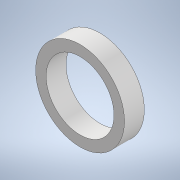
# Autodesk Inventor part: kokool
Saved by Autodesk Inventor 2022.3 (Build 263350000, 350)
## iProperties
Created: 2023-01-15
Part Number: kokool
Material: Generic
Document SubType Name: Modeling
Designer: komputer
Density: 1 g/cm^3
Appearance: Default
Author: komputer
Autodesk Inventor part; units mm, degrees
ref_plane "YZ Plane" through (0, 0, 0) normal (1, 0, 0) x (0, 1, 0)
ref_plane "XZ Plane" through (0, 0, 0) normal (0, 1, 0) x (-1, 0, 0)
ref_plane "XY Plane" through (0, 0, 0) normal (0, 0, 1) x (1, 0, 0)
sketch "Sketch1" plane through (0, 0, 0) normal (0, 0, 1) x (1, 0, 0)
  circle A0 centre (1.5, 0) radius 7 projected
  circle A1 centre (1.5, 0) radius 7 projected
  circle A2 centre (1.5, 0) radius 1.5 projected
  circle A3 centre (1.5, 0) radius 1 projected
  line L0 (16.2929, 8.3594) -> (-3.7046, 8.2678)
  line L1 (1.5, 0) -> (1.462, 8.2914)
  line L2 (1.462, 8.2914) -> (1.4574, 9.2914)
  line L3 (-7.6528, 0.7576) -> (-7.6612, 1.3735) projected
  ellipse E0 centre (-7.4913, -0.0469) end of major axis (-7.487, -1.0469) minor radius 0.015 projected
  ellipse E1 centre (-7.4913, -0.0469) end of major axis (-7.487, -1.0469) minor radius 0.015 projected
  ellipse E2 centre (-7.5641, 0.5606) end of major axis (-7.5648, 0.7606) minor radius 0.0029 (-7.5669, 0.6786) -> (-7.5649, 0.3868) ccw projected
  ellipse E3 centre (-7.607, -0.1095) end of major axis (-7.6033, -1.1095) minor radius 0.0145 projected
  ellipse E4 centre (-7.607, -0.1095) end of major axis (-7.6033, -1.1095) minor radius 0.0145 projected
  ellipse E5 centre (-7.4913, -0.0469) end of major axis (-7.487, -1.0469) minor radius 0.015 projected
  ellipse E6 centre (-7.4369, -0.2282) end of major axis (-7.4378, -0.0282) minor radius 0.003 (-7.4348, -0.4079) -> (-7.4361, -0.0582) ccw projected
  ellipse E7 centre (-7.4913, -0.0469) end of major axis (-7.487, -1.0469) minor radius 0.015 projected
  ellipse E8 centre (-7.4913, -0.0469) end of major axis (-7.487, -1.0469) minor radius 0.015 projected
  ellipse E9 centre (-7.5547, -1.7062) end of major axis (-7.5554, -1.5062) minor radius 0.0029 (-7.5538, -1.906) -> (-7.5527, -1.5926) ccw projected
  ellipse E10 centre (-7.6485, -1.6199) end of major axis (-7.6492, -1.4199) minor radius 0.0029 (-7.6512, -1.502) -> (-7.6479, -1.8195) ccw projected
  line L4 (-7.6369, -1.8711) -> (-7.6479, -1.8195) projected
  ellipse E11 centre (-7.6364, -2.0707) end of major axis (-7.6371, -1.8707) minor radius 0.0029 (-7.6334, -2.1069) -> (-7.6369, -1.8711) ccw projected
  line L5 (-7.6327, -2.8428) -> (-7.6334, -2.1069) projected
  ellipse E12 centre (-7.6297, -2.879) end of major axis (-7.6304, -2.679) minor radius 0.0029 (-7.6327, -2.8428) -> (-7.6279, -3.0648) ccw projected
  line L6 (-7.6189, -2.7874) -> (-7.6279, -3.0648) projected
  ellipse E13 centre (-7.6171, -2.9732) end of major axis (-7.6179, -2.7732) minor radius 0.0029 (-7.6145, -2.9205) -> (-7.6189, -2.7874) ccw projected
  line L7 (-7.609, -3.6423) -> (-7.6145, -2.9205) projected
  ellipse E14 centre (-7.6064, -3.5896) end of major axis (-7.6072, -3.3896) minor radius 0.0029 (-7.609, -3.6423) -> (-7.6038, -3.7248) ccw projected
  line L8 (-7.5985, -3.1734) -> (-7.6038, -3.7248) projected
  ellipse E15 centre (-7.5958, -3.3085) end of major axis (-7.5966, -3.1086) minor radius 0.0029 (-7.5941, -3.1773) -> (-7.5985, -3.1734) ccw projected
  line L9 (-7.585, -3.7421) -> (-7.5941, -3.1773) projected
  ellipse E16 centre (-7.5833, -3.6109) end of major axis (-7.584, -3.4109) minor radius 0.0029 (-7.585, -3.7421) -> (-7.5803, -3.6688) ccw projected
  line L10 (-7.5798, -2.9524) -> (-7.5803, -3.6688) projected
  ellipse E17 centre (-7.5768, -3.0103) end of major axis (-7.5775, -2.8103) minor radius 0.0029 (-7.5763, -2.8266) -> (-7.5798, -2.9524) ccw projected
  line L11 (-7.5652, -3.1224) -> (-7.5763, -2.8266) projected
  ellipse E18 centre (-7.5648, -2.9387) end of major axis (-7.5655, -2.7387) minor radius 0.0029 (-7.5652, -3.1224) -> (-7.562, -2.9078) ccw projected
  line L12 (-7.5664, -2.1685) -> (-7.562, -2.9078) projected
  ellipse E19 centre (-7.5637, -2.1375) end of major axis (-7.5644, -1.9375) minor radius 0.0029 (-7.5645, -1.9377) -> (-7.5664, -2.1685) ccw projected
  line L13 (-7.5538, -1.906) -> (-7.5645, -1.9377) projected
  ellipse E20 centre (-7.5547, -1.7062) end of major axis (-7.5554, -1.5062) minor radius 0.0029 (-7.5538, -1.906) -> (-7.5527, -1.5926) ccw projected
  line L14 (-7.5611, -0.9767) -> (-7.5527, -1.5926) projected
  ellipse E21 centre (-7.5591, -0.8631) end of major axis (-7.5599, -0.6631) minor radius 0.0029 (-7.5612, -0.6867) -> (-7.5611, -0.9767) ccw projected
  line L15 (-7.5529, -0.3338) -> (-7.5612, -0.6867) projected
  ellipse E22 centre (-7.5549, -0.1574) end of major axis (-7.5556, 0.0426) minor radius 0.0029 (-7.5529, -0.3338) -> (-7.5541, 0.0164) ccw projected
  line L16 (-7.5649, 0.3868) -> (-7.5541, 0.0164) projected
  ellipse E23 centre (-7.5641, 0.5606) end of major axis (-7.5648, 0.7606) minor radius 0.0029 (-7.5669, 0.6786) -> (-7.5649, 0.3868) ccw projected
  line L17 (-7.5627, 1.2829) -> (-7.5669, 0.6786) projected
  ellipse E24 centre (-7.5655, 1.4008) end of major axis (-7.5662, 1.6008) minor radius 0.0029 (-7.5627, 1.2829) -> (-7.566, 1.6004) ccw projected
  line L18 (-7.577, 1.652) -> (-7.566, 1.6004) projected
  ellipse E25 centre (-7.5775, 1.8516) end of major axis (-7.5783, 2.0516) minor radius 0.0029 (-7.5805, 1.8878) -> (-7.577, 1.652) ccw projected
  line L19 (-7.5812, 2.6237) -> (-7.5805, 1.8878) projected
  ellipse E26 centre (-7.5842, 2.66) end of major axis (-7.585, 2.86) minor radius 0.0029 (-7.5812, 2.6237) -> (-7.586, 2.8457) ccw projected
  line L20 (-7.595, 2.5683) -> (-7.586, 2.8457) projected
  ellipse E27 centre (-7.5968, 2.7541) end of major axis (-7.5975, 2.9541) minor radius 0.0029 (-7.5994, 2.7014) -> (-7.595, 2.5683) ccw projected
  line L21 (-7.6049, 3.4233) -> (-7.5994, 2.7014) projected
  ellipse E28 centre (-7.6075, 3.3705) end of major axis (-7.6082, 3.5705) minor radius 0.0029 (-7.6049, 3.4233) -> (-7.6101, 3.5057) ccw projected
  line L22 (-7.6154, 2.9543) -> (-7.6101, 3.5057) projected
  ellipse E29 centre (-7.6181, 3.0895) end of major axis (-7.6188, 3.2895) minor radius 0.0029 (-7.6198, 2.9582) -> (-7.6154, 2.9543) ccw projected
  line L23 (-7.629, 3.523) -> (-7.6198, 2.9582) projected
  ellipse E30 centre (-7.6307, 3.3918) end of major axis (-7.6314, 3.5918) minor radius 0.0029 (-7.629, 3.523) -> (-7.6337, 3.4497) ccw projected
  line L24 (-7.6342, 2.7334) -> (-7.6337, 3.4497) projected
  ellipse E31 centre (-7.6372, 2.7912) end of major axis (-7.6379, 2.9912) minor radius 0.0029 (-7.6376, 2.6075) -> (-7.6342, 2.7334) ccw projected
  line L25 (-7.6487, 2.9034) -> (-7.6376, 2.6075) projected
  ellipse E32 centre (-7.6492, 2.7196) end of major axis (-7.6499, 2.9196) minor radius 0.0029 (-7.6487, 2.9034) -> (-7.6519, 2.6887) ccw projected
  line L26 (-7.6475, 1.9494) -> (-7.6519, 2.6887) projected
  ellipse E33 centre (-7.6503, 1.9184) end of major axis (-7.651, 2.1184) minor radius 0.0029 (-7.6494, 1.7186) -> (-7.6475, 1.9494) ccw projected
  line L27 (-7.6601, 1.6869) -> (-7.6494, 1.7186) projected
  ellipse E34 centre (-7.6593, 1.4871) end of major axis (-7.66, 1.6871) minor radius 0.0029 (-7.6601, 1.6869) -> (-7.6612, 1.3735) ccw projected
  line L28 (-7.6528, 0.7576) -> (-7.6612, 1.3735) projected
  ellipse E35 centre (-7.6548, 0.644) end of major axis (-7.6555, 0.844) minor radius 0.0029 (-7.6528, 0.4676) -> (-7.6528, 0.7576) ccw projected
  line L29 (-7.661, 0.1147) -> (-7.6528, 0.4676) projected
  ellipse E36 centre (-7.659, -0.0617) end of major axis (-7.6598, 0.1383) minor radius 0.0029 (-7.661, 0.1147) -> (-7.6598, -0.2354) ccw projected
  line L30 (-7.649, -0.6059) -> (-7.6598, -0.2354) projected
  ellipse E37 centre (-7.6498, -0.7797) end of major axis (-7.6506, -0.5797) minor radius 0.0029 (-7.6471, -0.8977) -> (-7.649, -0.6059) ccw projected
  line L31 (-7.6512, -1.502) -> (-7.6471, -0.8977) projected
  ellipse E38 centre (-7.6485, -1.6199) end of major axis (-7.6492, -1.4199) minor radius 0.0029 (-7.6512, -1.502) -> (-7.6479, -1.8195) ccw projected
  ellipse E39 centre (-7.6485, -1.6199) end of major axis (-7.6492, -1.4199) minor radius 0.0029 (-7.6512, -1.502) -> (-7.6479, -1.8195) ccw projected
  line L32 (-7.5611, -0.9767) -> (-7.5527, -1.5926) projected
  line L33 (-7.5611, -0.9767) -> (-7.5527, -1.5926) projected
  line L34 (-7.5611, -0.9767) -> (-7.5527, -1.5926) projected
  line L35 (-7.5611, -0.9767) -> (-7.5527, -1.5926) projected
  ellipse E40 centre (-7.6498, -0.7797) end of major axis (-7.6506, -0.5797) minor radius 0.0029 (-7.6471, -0.8977) -> (-7.649, -0.6059) ccw projected
  ellipse E41 centre (-7.607, -0.1095) end of major axis (-7.6033, -1.1095) minor radius 0.0145 projected
  line L36 (-7.661, 0.1147) -> (-7.6528, 0.4676) projected
  ellipse E42 centre (-7.5655, 1.4008) end of major axis (-7.5662, 1.6008) minor radius 0.0029 (-7.5627, 1.2829) -> (-7.566, 1.6004) ccw projected
  line L37 (-7.5335, 2.0955) -> (-7.538, 2.8386) projected
  line L38 (-7.5812, 2.6237) -> (-7.5805, 1.8878) projected
  line L39 (-7.5335, 2.0955) -> (-7.538, 2.8386) projected
  ellipse E43 centre (-7.5363, 2.072) end of major axis (-7.5372, 2.272) minor radius 0.003 (-7.5355, 1.872) -> (-7.5335, 2.0955) ccw projected
  line L40 (-7.5467, 1.8682) -> (-7.5355, 1.872) projected
  ellipse E44 centre (-7.5458, 1.6682) end of major axis (-7.5466, 1.8682) minor radius 0.003 (-7.5467, 1.8682) -> (-7.5478, 1.5608) ccw projected
  line L41 (-7.5391, 0.9295) -> (-7.5478, 1.5608) projected
  ellipse E45 centre (-7.5412, 0.8221) end of major axis (-7.542, 1.0221) minor radius 0.003 (-7.5391, 0.6423) -> (-7.5391, 0.9295) ccw projected
  line L42 (-7.5477, 0.3142) -> (-7.5391, 0.6423) projected
  ellipse E46 centre (-7.5456, 0.1345) end of major axis (-7.5465, 0.3345) minor radius 0.003 (-7.5477, 0.3142) -> (-7.5465, -0.0355) ccw projected
  line L43 (-7.5352, -0.43) -> (-7.5465, -0.0355) projected
  ellipse E47 centre (-7.5361, -0.5999) end of major axis (-7.5369, -0.3999) minor radius 0.003 (-7.5332, -0.7238) -> (-7.5352, -0.43) ccw projected
  line L44 (-7.5376, -1.3113) -> (-7.5332, -0.7238) projected
  ellipse E48 centre (-7.5347, -1.4352) end of major axis (-7.5356, -1.2352) minor radius 0.003 (-7.5376, -1.3113) -> (-7.5342, -1.634) ccw projected
  line L45 (-7.5227, -1.7135) -> (-7.5342, -1.634) projected
  ellipse E49 centre (-7.5221, -1.9124) end of major axis (-7.523, -1.7124) minor radius 0.003 (-7.519, -1.9559) -> (-7.5227, -1.7135) ccw projected
  line L46 (-7.5183, -2.6863) -> (-7.519, -1.9559) projected
  ellipse E50 centre (-7.5152, -2.7298) end of major axis (-7.5161, -2.5298) minor radius 0.003 (-7.5183, -2.6863) -> (-7.5134, -2.9182) ccw projected
  line L47 (-7.5039, -2.6669) -> (-7.5134, -2.9182) projected
  ellipse E51 centre (-7.5021, -2.8553) end of major axis (-7.5029, -2.6553) minor radius 0.003 (-7.4994, -2.8098) -> (-7.5039, -2.6669) ccw projected
  line L48 (-7.4937, -3.5386) -> (-7.4994, -2.8098) projected
  ellipse E52 centre (-7.4909, -3.4931) end of major axis (-7.4918, -3.2931) minor radius 0.003 (-7.4937, -3.5386) -> (-7.4882, -3.6337) ccw projected
  line L49 (-7.4826, -3.1014) -> (-7.4882, -3.6337) projected
  ellipse E53 centre (-7.4799, -3.242) end of major axis (-7.4808, -3.042) minor radius 0.003 (-7.4781, -3.1166) -> (-7.4826, -3.1014) ccw projected
  line L50 (-7.4685, -3.6993) -> (-7.4781, -3.1166) projected
  ellipse E54 centre (-7.4668, -3.5738) end of major axis (-7.4676, -3.3738) minor radius 0.003 (-7.4685, -3.6993) -> (-7.4636, -3.6387) ccw projected
  line L51 (-7.4631, -2.9309) -> (-7.4636, -3.6387) projected
  ellipse E55 centre (-7.4599, -2.9959) end of major axis (-7.4608, -2.7959) minor radius 0.003 (-7.4594, -2.8153) -> (-7.4631, -2.9309) ccw projected
  line L52 (-7.4479, -3.1365) -> (-7.4594, -2.8153) projected
  ellipse E56 centre (-7.4474, -2.9559) end of major axis (-7.4483, -2.7559) minor radius 0.003 (-7.4479, -3.1365) -> (-7.4446, -2.9324) ccw projected
  line L53 (-7.4491, -2.1892) -> (-7.4446, -2.9324) projected
  ellipse E57 centre (-7.4462, -2.1657) end of major axis (-7.4471, -1.9657) minor radius 0.003 (-7.4471, -1.9657) -> (-7.4491, -2.1892) ccw projected
  line L54 (-7.4359, -1.9619) -> (-7.4471, -1.9657) projected
  ellipse E58 centre (-7.4368, -1.7619) end of major axis (-7.4376, -1.5619) minor radius 0.003 (-7.4359, -1.9619) -> (-7.4347, -1.6545) ccw projected
  line L55 (-7.4435, -1.0232) -> (-7.4347, -1.6545) projected
  ellipse E59 centre (-7.4414, -0.9158) end of major axis (-7.4423, -0.7158) minor radius 0.003 (-7.4435, -0.736) -> (-7.4435, -1.0232) ccw projected
  line L56 (-7.4348, -0.4079) -> (-7.4435, -0.736) projected
  ellipse E60 centre (-7.4369, -0.2282) end of major axis (-7.4378, -0.0282) minor radius 0.003 (-7.4348, -0.4079) -> (-7.4361, -0.0582) ccw projected
  line L57 (-7.4473, 0.3362) -> (-7.4361, -0.0582) projected
  ellipse E61 centre (-7.4465, 0.5062) end of major axis (-7.4473, 0.7062) minor radius 0.003 (-7.4494, 0.6301) -> (-7.4473, 0.3362) ccw projected
  line L58 (-7.445, 1.2175) -> (-7.4494, 0.6301) projected
  ellipse E62 centre (-7.4478, 1.3414) end of major axis (-7.4487, 1.5414) minor radius 0.003 (-7.445, 1.2175) -> (-7.4484, 1.5403) ccw projected
  line L59 (-7.4599, 1.6198) -> (-7.4484, 1.5403) projected
  ellipse E63 centre (-7.4604, 1.8186) end of major axis (-7.4613, 2.0186) minor radius 0.003 (-7.4635, 1.8622) -> (-7.4599, 1.6198) ccw projected
  line L60 (-7.4642, 2.5926) -> (-7.4635, 1.8622) projected
  ellipse E64 centre (-7.4674, 2.6361) end of major axis (-7.4682, 2.8361) minor radius 0.003 (-7.4642, 2.5926) -> (-7.4692, 2.8245) ccw projected
  line L61 (-7.4787, 2.5732) -> (-7.4692, 2.8245) projected
  ellipse E65 centre (-7.4805, 2.7616) end of major axis (-7.4813, 2.9616) minor radius 0.003 (-7.4832, 2.7161) -> (-7.4787, 2.5732) ccw projected
  line L62 (-7.4889, 3.4448) -> (-7.4832, 2.7161) projected
  ellipse E66 centre (-7.4916, 3.3993) end of major axis (-7.4925, 3.5993) minor radius 0.003 (-7.4889, 3.4448) -> (-7.4944, 3.5399) ccw projected
  line L63 (-7.4999, 3.0077) -> (-7.4944, 3.5399) projected
  ellipse E67 centre (-7.5027, 3.1483) end of major axis (-7.5035, 3.3483) minor radius 0.003 (-7.5045, 3.0228) -> (-7.4999, 3.0077) ccw projected
  line L64 (-7.514, 3.6055) -> (-7.5045, 3.0228) projected
  ellipse E68 centre (-7.5158, 3.48) end of major axis (-7.5167, 3.68) minor radius 0.003 (-7.514, 3.6055) -> (-7.5189, 3.545) ccw projected
  line L65 (-7.5195, 2.8372) -> (-7.5189, 3.545) projected
  ellipse E69 centre (-7.5226, 2.9022) end of major axis (-7.5235, 3.1022) minor radius 0.003 (-7.5231, 2.7216) -> (-7.5195, 2.8372) ccw projected
  line L66 (-7.5346, 3.0428) -> (-7.5231, 2.7216) projected
  ellipse E70 centre (-7.5351, 2.8622) end of major axis (-7.536, 3.0622) minor radius 0.003 (-7.5346, 3.0428) -> (-7.538, 2.8386) ccw projected
  line L67 (-5.5, -0.0031) -> (-7.664, -0.0125)
  circle A4 centre (1.5, 0) radius 9.164
  point P0 (0, 0)
  dimension "d0" = 1
  constraints: 8 end point, 2 point on line, 1 coincident, 1 horizontal alignment, 1 perpendicular, 72 other
  measures "d0" distance of L1.end L2.end
extrude "Extrusion1" add sketch "Sketch1" along normal blind 2.5 contours A0 | L67 L57 E61 L58 E62 L59 E63 L60 A4 L0 L1 A0 | A0 L1 L0 A4 E57 L54 E58 L55 E59 L56 E6 L57 L67 | L67 E0 E46 L42 E45 L41 A4 L60 E63 L59 E62 L58 E61 L57 | L57 E6 L56 E59 L55 E58 L54 E57 A4 E3 L67 E0 | L2 A4 L0 | L0 A4 L2 | L67 E0 | E0 L67 | A4 L29 E36 | L67 E22 L16 E2 L17 E24 A4 L41 E45 L42 E46 | L67 E3 E36 L29 A4 E24 L17 E2 L16 E22 | L67 E3 | E3 A4 L67 | E3 A4 E36 L67 | A2 | A3
sketch "Sketch2" plane through (1.5, 0, 0) normal (0, 0, -1) x (-1, 0, 0)
  circle A0 centre (0, 0) radius 9.164 projected
  circle A1 centre (0, 0) radius 7 projected
  point P0 (1.5, 0)
extrude "Extrusion2" add sketch "Sketch2" along normal blind 2
sketch "Sketch3" plane through (1.5, 0, 2.5) normal (0, 0, 1) x (1, 0, 0)
  circle A0 centre (0, 0) radius 7 projected
  point P0 (-1.5, 0)
extrude "Extrusion3" cut sketch "Sketch3" against normal through all
sketch "Sketch4" plane through (1.5, 0, 2.5) normal (0, 0, 1) x (1, 0, 0)
  circle A0 centre (0, 0) radius 7 projected
  circle A1 centre (0, 0) radius 9.164 projected
  point P0 (-1.5, 0)
extrude "Extrusion4" cut sketch "Sketch4" against normal blind 0.4
body "Solid1"
